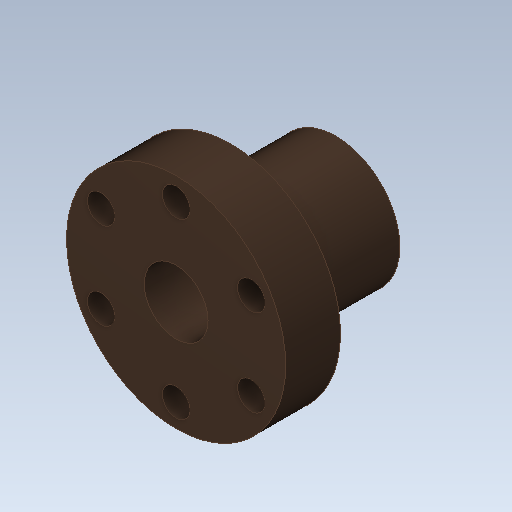
# Autodesk Inventor part: Cartesian1_Z_TrapezoiadlNut
Saved by Autodesk Inventor 2020 (Build 240168000, 168)
## iProperties
Created: 2020-03-02
Part Number: Cartesian1_Z_TrapezoiadlNut
Material: Brąz, miękki cynowy
Document SubType Name: Modeling
Designer: invin
Density: 8.874 g/cm^3
Appearance: Brąz — satynowy
Mass: 252.496 g
Surface Area: 97.0124 cm^2
Volume: 28.4534 cm^3
Author: invin
Autodesk Inventor part; units mm, degrees
ref_plane "YZ Plane" through (0, 0, 0) normal (1, 0, 0) x (0, 1, 0)
ref_plane "XZ Plane" through (0, 0, 0) normal (0, 1, 0) x (-1, 0, 0)
ref_plane "XY Plane" through (0, 0, 0) normal (0, 0, 1) x (1, 0, 0)
sketch "Szkic1" plane through (0, 0, 0) normal (0, 0, 1) x (1, 0, 0)
  circle A0 centre (0, 0) radius 24
  circle A1 centre (0, 0) radius 14
  dimension "d0" = 48
  dimension "d1" = 28
  constraints: 2 centre point, 2 coincident
  measures "d0" diameter of A0
  measures "d1" diameter of A1
extrude "Wyciągnięcie proste1" add sketch "Szkic1" along normal blind 12
sketch "Szkic2" plane through (0, 0, 12) normal (0, 0, 1) x (1, 0, 0)
  circle A0 centre (0, 0) radius 19
  circle A1 centre (0, 19) radius 3
  dimension "d4" = 38
  dimension "d5" = 6
  constraints: 1 centre point, 1 coincident, 1 vertical alignment, 2 other
  measures "d5" diameter of A1
extrude "Wyciągnięcie proste2" cut sketch "Szkic2" against normal blind 12 contours A1 A0 | A0 A1 picked at (0, 17.9824) picked at (0.0843, 19.9789)
pattern_circular "Szyk kołowy1" count 6 over 360 about axis through (0, 0, 0) along (0, 0, 1) of "Wyciągnięcie proste2"
sketch "Szkic3" plane through (0, 0, 12) normal (0, 0, 1) x (1, 0, 0)
  circle A0 centre (0, 0) radius 14
  circle A1 centre (0, 0) radius 7
  dimension "d11" = 28
  dimension "d12" = 14
  constraints: 2 centre point, 2 coincident
  measures "d11" diameter of A0
  measures "d12" diameter of A1
extrude "Wyciągnięcie proste3" add sketch "Szkic3" against normal blind 35
